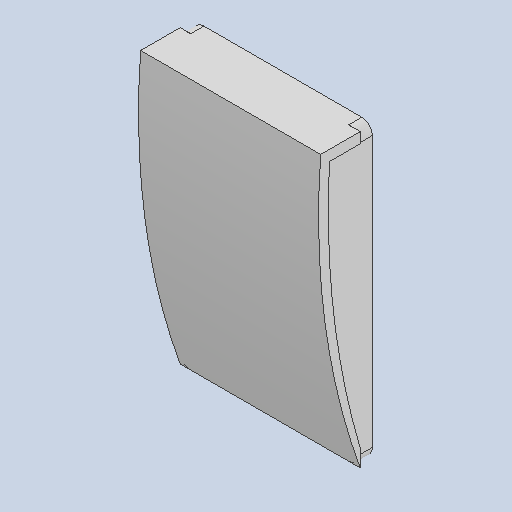
# Autodesk Inventor part: krish
Saved by Autodesk Inventor 2022 (Build 260153000, 153)
## iProperties
Created: 2023-05-24
Part Number: krish
Material: Типовые
Document SubType Name: Modeling
Designer: korsh624
Density: 1 g/cm^3
Appearance: По умолчанию
Author: korsh624
Autodesk Inventor part; units mm, degrees
ref_plane "YZ Plane" through (0, 0, 0) normal (1, 0, 0) x (0, 1, 0)
ref_plane "XZ Plane" through (0, 0, 0) normal (0, 1, 0) x (-1, 0, 0)
ref_plane "XY Plane" through (0, 0, 0) normal (0, 0, 1) x (1, 0, 0)
sketch "Эскиз1" plane through (0, 0, 0) normal (0, 0, 1) x (1, 0, 0)
  line L0 (5, 13) -> (5, 207.8488) projected
  arc A0 (13, 215.8488) -> (5, 207.8488) centre (13, 207.8488) ccw projected
  line L1 (13, 215.8488) -> (122.6512, 215.8488) projected
  arc A1 (130.6512, 207.8488) -> (122.6512, 215.8488) centre (122.6512, 207.8488) ccw projected
  line L2 (130.6512, 207.8488) -> (130.6512, 13) projected
  arc A2 (122.6512, 5) -> (130.6512, 13) centre (122.6512, 13) ccw projected
  line L3 (13, 5) -> (122.6512, 5) projected
  arc A3 (5, 13) -> (13, 5) centre (13, 13) ccw projected
  arc A4 (127.6512, 0) -> (135.6512, 8) centre (127.6512, 8) ccw projected
  line L4 (135.6512, 8) -> (135.6512, 212.8488) projected
  arc A5 (135.6512, 212.8488) -> (127.6512, 220.8488) centre (127.6512, 212.8488) ccw projected
  line L5 (127.6512, 220.8488) -> (8, 220.8488) projected
  arc A6 (8, 220.8488) -> (0, 212.8488) centre (8, 212.8488) ccw projected
  line L6 (0, 8) -> (0, 212.8488) projected
  arc A7 (0, 8) -> (8, 0) centre (8, 8) ccw projected
  line L7 (127.6512, 0) -> (8, 0) projected
  point P0 (0, 0)
extrude "Выдавливание1" add sketch "Эскиз1" along normal blind 10
sketch "Эскиз2" plane through (0, 8, 0) normal (-1, 0, 0) x (0, 0, 1)
  line L0 (0, 212.8488) -> (10, 212.8488) projected
  line L1 (10, 212.8488) -> (40, 212.8488)
  arc A0 (10, -8) -> (40, 212.8488) centre (-486.9233, 171.9638) ccw
  line L2 (10, 212.8488) -> (10, -8)
  line L3 (10, 5) -> (10, -3) projected
  arc A1 (10, 5) -> (32.8436, 212.8488) centre (-556.7291, 172.466) ccw
  line L4 (0, 204.8488) -> (10, 204.8488) projected
  line L5 (10, 204.8488) -> (33.3371, 204.8488)
  point P0 (0, -8)
  dimension "d2" = 30
  constraints: 6 end point, 5 point on circle, 2 centre point, 2 collinear, 1 horizontal, 1 point on line
  measures "d2" distance of L0.end L1.end
extrude "Выдавливание2" add sketch "Эскиз2" against normal blind 136.5 contours L1 A1 L5 L2 | L1 A0 L2 A1
sketch "Эскиз3" plane through (135.6512, 8, 0) normal (1, 0, 0) x (0, 0, -1)
  line L0 (-10, 5) -> (-10, 204.8488) projected
  arc A0 (-33.3371, 204.8488) -> (-10, 5) centre (556.7291, 172.466) ccw projected
  line L1 (-33.3371, 204.8488) -> (-10, 204.8488) projected
  point P0 (0, -8)
extrude "Выдавливание3" add sketch "Эскиз3" against normal blind 5
sketch "Эскиз4" plane through (0, 8, 0) normal (-1, 0, 0) x (0, 0, 1)
  arc A0 (10, 5) -> (33.3371, 204.8488) centre (-556.7291, 172.466) ccw projected
  line L0 (10, 204.8488) -> (10, 5) projected
  line L1 (10, 204.8488) -> (33.3371, 204.8488) projected
  point P0 (0, -8)
extrude "Выдавливание4" add sketch "Эскиз4" against normal blind 5
